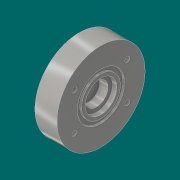
# Autodesk Inventor part: .5 in hole
Saved by Autodesk Inventor 2016 (Build 200138000, 138)
## iProperties
Created: 2016-06-27
Part Number: .5 in hole
Material: Aluminum 6061
Document SubType Name: Modeling
Designer: Jonathan
Density: 2.7 g/cm^3
Appearance: Aluminum - Polished
Author: Jonathan
Autodesk Inventor part; units mm, degrees
ref_plane "YZ Plane" through (0, 0, 0) normal (1, 0, 0) x (0, 1, 0)
ref_plane "XZ Plane" through (0, 0, 0) normal (0, 1, 0) x (-1, 0, 0)
ref_plane "XY Plane" through (0, 0, 0) normal (0, 0, 1) x (1, 0, 0)
sketch "Sketch1" plane through (0, 0, 0) normal (1, 0, 0) x (0, 1, 0)
  circle A0 centre (0, 0) radius 25.4
  dimension "d0" = 50.8
  constraints: 1 centre point, 1 coincident
  measures "d0" diameter of A0
extrude "Extrusion1" add sketch "Sketch1" along normal blind 12.7
sketch "Sketch10" plane through (12.7, 0, 0) normal (1, 0, 0) x (0, 0, -1)
  point P0 (0, 0)
  point P1 (0, 0)
  constraints: 1 coincident
hole "Hole4" at (12.7, 0, 0) direction (-1, 0, 0) diameter 18.2563 depth 2.54
sketch "Sketch11" plane through (10.16, 0, 0) normal (1, 0, 0) x (0, 0, -1)
  point P0 (0, 0)
  point P1 (0, 0)
  constraints: 1 coincident
hole "Hole7" at (10.16, 0, 0) direction (-1, 0, 0) diameter 13.0969 depth 4.7625
sketch "Sketch12" plane through (0, 0, 0) normal (-1, 0, 0) x (0, 0, 1)
  line L0 (-10.795, 15.24) -> (10.795, 15.24) construction
  line L1 (10.795, 15.24) -> (10.795, -15.24) construction
  line L2 (10.795, -15.24) -> (-10.795, -15.24) construction
  line L3 (-10.795, -15.24) -> (-10.795, 15.24) construction
  line L4 (-10.795, 15.24) -> (10.795, -15.24) construction
  line L5 (10.795, 15.24) -> (-10.795, -15.24) construction
  point P0 (0, 0)
  dimension "d107" = 21.59
  dimension "d108" = 30.48
  constraints: 12 end point, 4 coincident, 2 midpoint, 2 parallel, 1 horizontal, 1 perpendicular
  measures "d107" distance of L1.end L2.end
  measures "d108" distance of L0.end L1.end
hole "Hole8" at (0, 15.24, 10.795) at (0, -15.24, 10.795) at (0, -15.24, -10.795) at (0, 15.24, -10.795) direction (1, 0, 0) diameter 2.9464 end through all clearance for "Socket Head Cap Screw" size "#4" standard "Ansi Unified Screw Threads"
sketch "Sketch13" plane through (0, 0, 0) normal (-1, 0, 0) x (0, 0, 1)
  point P0 (0, 0)
  point P1 (0, 0)
  constraints: 1 coincident
hole "Hole9" at (0, 0, 0) direction (1, 0, 0) diameter 1 end through all
sketch "Sketch9" plane through (0, 0, 0) normal (0, 1, 0) x (-1, 0, 0)
  line L0 (-11.4554, -11.1252) -> (-12.7, -11.1252)
  line L1 (-12.7, -11.1252) -> (-12.7, -13.6652)
  line L2 (-12.7, -13.6652) -> (-11.4554, -13.6652)
  line L3 (-11.4554, -13.6652) -> (-11.4554, -11.1252)
  line L4 (2.54, 0) -> (-15.24, 0) projected
  line L5 (-12.7, 25.4) -> (-12.7, -25.4) projected
  point P0 (0, 0)
  dimension "d55" = 2.54
  dimension "d56" = 1.2446
  dimension "d59" = 11.1252
  constraints: 8 end point, 2 parallel, 1 collinear, 1 perpendicular
  measures "d55" distance of L2.end L0.start
  measures "d56" distance of L1.end L2.end
  measures "d59" distance between parallel lines of L4 L0
revolve "Revolution1" cut sketch "Sketch9" angle 360 about axis through (-10, 0, 0) along (1, 0, 0)
sketch "Sketch14" plane through (0, 0, 0) normal (-1, 0, 0) x (0, 0, 1)
  line L0 (-9.5, 0) -> (9.5, 0)
  circle A0 centre (0, 0) radius 0.5 projected
  dimension "d123" = 19
  dimension "d124" = 9.5
  constraints: 2 end point, 1 horizontal, 1 midpoint
  measures "d123" distance of L0.end L0.start
  measures "d124" distance of A0.centre L0.start
hole "Hole10" at (0, 0, 9.5) at (0, 0, -9.5) direction (1, 0, 0) diameter 2.159 depth 8.8646 tip angle 118
equation "\"d0\" = sensorHolderDiameter"
equation "\"d1\" = sensorHolderThickness"
equation "\"d100\" = glassTubeDiameter + 2 * glassTubeClearance"
equation "\"d107\" = shortHoleSpacing"
equation "\"d108\" = longHoleSpacing"
equation "\"d116\" = fiberDiameter + 2 * fiberClearance"
equation "\"d55\" = oRingGrooveWidth"
equation "\"d56\" = oRingGrooveDepth"
equation "\"d59\" = 0.5 * oRingID"
equation "\"d123\" = sensorBoardHoleSpacing"
equation "\"d124\" = 0.5 * d123"
equation "\"tubeHeight\" = 50.8"
equation "\"tubeWidth\" = 152.4"
equation "\"tubeLength\" = 304.8"
equation "\"tubeWallThickness\" = 3.175"
equation "\"plateOverhang\" = 6.35"
equation "\"moatWidth\" = 3.175"
equation "\"moatDepth\" = 3.175"
equation "\"tubePlateClearance\" = 0.127"
equation "\"blankCapThickness\" = 9.525"
equation "\"sensorCapThickness\" = 12.7"
equation "\"glassTubeDiameter\" = 12.7"
equation "\"glassTubeClearance\" = 0.19844"
equation "\"longHoleSpacing\" = 30.48"
equation "\"shortHoleSpacing\" = 21.59"
equation "\"sensorHolderDiameter\" = 50.8"
equation "\"sensorHolderThickness\" = 12.7"
equation "\"fiberClearence\" = 0"
equation "\"fiberDiameter\" = 1"
equation "\"fiberClearance\" = 0"
equation "\"oRingGrooveDepth\" = 1.2446"
equation "\"oRingGrooveWidth\" = 2.54"
equation "\"oRingID\" = 22.2504"
equation "\"glassTubeLength\" = 279.4"
equation "\"glassTubeID\" = 7.874"
equation "\"sensorBoardHoleSpacing\" = 19"
body "Solid1"
